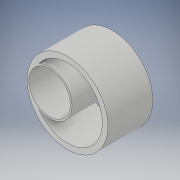
# Autodesk Inventor part: RO mark final
Saved by Autodesk Inventor 2019 (Build 230136000, 136)
## iProperties
Created: 2019-10-19
Part Number: RO mark final
Material: Generic
Document SubType Name: Modeling
Designer: Connor Duggan
Density: 1 g/cm^3
Appearance: Default
Author: Connor Duggan
Autodesk Inventor part; units mm, degrees
ref_plane "YZ Plane" through (0, 0, 0) normal (1, 0, 0) x (0, 1, 0)
ref_plane "XZ Plane" through (0, 0, 0) normal (0, 1, 0) x (-1, 0, 0)
ref_plane "XY Plane" through (0, 0, 0) normal (0, 0, 1) x (1, 0, 0)
sketch "Sketch1" plane through (0, 0, 0) normal (0, 0, 1) x (1, 0, 0)
  line L0 (-6.35, 0) -> (-14.7828, 0) construction
  line L1 (0, 0) -> (30.9372, 0) construction
  circle A0 centre (30.9372, 0) radius 45.72
  line L2 (-14.7828, 0) -> (10.6172, 0) construction
  arc A1 (-1.4875, -22.3302) -> (-1.4875, 22.3302) centre (10.6172, 0) ccw
  arc A2 (-3.7794, -18.5675) -> (-3.7794, 18.5675) centre (10.6172, 0) ccw
  arc A3 (-1.4875, -22.3302) -> (-1.4875, 22.3302) centre (30.9372, 0) ccw
  arc A4 (-3.7794, 18.5675) -> (-3.7794, -18.5675) centre (10.6172, 0) ccw
  dimension "d1" = 8.4328
  dimension "d2" = 30.9372
  dimension "d6" = 25.4
  dimension "d7" = 46.99
  constraints: 8 point on circle, 6 end point, 5 coincident, 4 centre point, 2 horizontal, 1 horizontal alignment, 1 point on line, 2 other
  measures "d1" distance of L0.start L0.end
  measures "d2" distance of L1.start L1.end
  measures "d6" distance of L0.end L2.end
  measures "d7" diameter of A2
extrude "Extrusion1" add sketch "Sketch1" along normal blind 50.8
body "Solid1"
